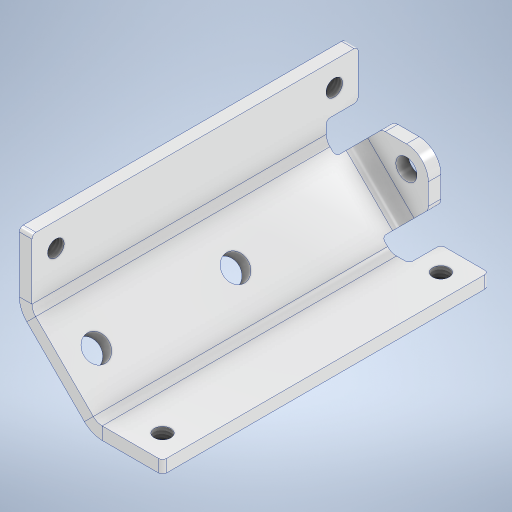
# Autodesk Inventor part: Exterior Frame Gantry Brace
Saved by Autodesk Inventor 2024 (Build 280153000, 153)
## iProperties
Created: 2024-12-02
Part Number: Exterior Frame Gantry Brace
Material: Aluminum 6061
Document SubType Name: Sheet Metal
Designer: Ishaan
Density: 2.7 g/cm^3
Sheet Metal Rule: SendCutSend_1-8_Alu
Appearance: Aluminum - Flat
Author: Ishaan
Autodesk Inventor part; units mm, degrees
ref_plane "YZ Plane" through (0, 0, 0) normal (1, 0, 0) x (0, 1, 0)
ref_plane "XZ Plane" through (0, 0, 0) normal (0, 1, 0) x (-1, 0, 0)
ref_plane "XY Plane" through (0, 0, 0) normal (0, 0, 1) x (1, 0, 0)
sketch "Sketch1" plane through (0, 0, 0) normal (0, 0, 1) x (1, 0, 0)
  line L0 (0, -21.2132) -> (-21.2132, 0) construction
  line L1 (-21.2132, 0) -> (0, 21.2132) construction
  line L2 (0, 21.2132) -> (21.2132, 0) construction
  line L3 (21.2132, 0) -> (0, -21.2132) construction
  line L4 (0, -21.2132) -> (0, 21.2132) construction
  line L5 (-21.2132, 0) -> (21.2132, 0) construction
  line L6 (42.4264, -1.5) -> (0, -1.5) construction
  line L7 (0, -1.5) -> (0, 1.5) construction
  line L8 (0, 1.5) -> (42.4264, 1.5) construction
  line L9 (42.4264, 1.5) -> (42.4264, -1.5) construction
  line L10 (42.4264, -1.5) -> (0, 1.5) construction
  line L11 (0, -1.5) -> (42.4264, 1.5) construction
  line L12 (-1.5, 42.4264) -> (1.5, 42.4264) construction
  line L13 (1.5, 42.4264) -> (1.5, 0) construction
  line L14 (1.5, 0) -> (-1.5, 0) construction
  line L15 (-1.5, 0) -> (-1.5, 42.4264) construction
  line L16 (-1.5, 42.4264) -> (1.5, 0) construction
  line L17 (1.5, 42.4264) -> (-1.5, 0) construction
  line L18 (31.5, 1.5) -> (31.5, -7.4041) construction
  line L19 (1.5, 31.5) -> (-12.6446, 31.5) construction
  line L20 (24, 1.5) -> (24, -1.5) construction
  line L21 (37.5, 1.5) -> (19.7132, 1.5)
  line L22 (19.7132, 1.5) -> (1.5, 19.7132)
  line L23 (1.5, 19.7132) -> (1.5, 37.5)
  point P0 (0, 0)
  point P1 (0, 0)
  point P2 (0, 0)
  point P3 (0, 0)
  dimension "d0" = 30
  dimension "d1" = 3
  dimension "d2" = 3
  dimension "d4" = 31.5
  dimension "d5" = 31.5
  dimension "d6" = 24
  dimension "d7" = 7.5
  dimension "d18" = 6
  dimension "d19" = 6
  measures "d0" distance of L0.end L1.end
  measures "d1" distance of L6.end L7.end
  measures "d2" distance of L13.end L14.end
  measures "d4" distance from line of L18 point (0, 0)
  measures "d5" distance from line of point (0, 0) L19
  measures "d6" distance from line of point (0, 0) L20
  measures "d7" distance between parallel lines of L20 L18
  measures "d18" distance from line of L23.end L19
  measures "d19" distance from line of L21.start L18
contour flange "Contour Flange1" sketch "Sketch1" thickness 3.175 bend radius 3.175 width 82 along (0, 0, 1) mid plane no both sides no wall seen from (28.6066, 1.5, 0) lies toward (0, 1, 0) curves L21 L22 L23
bend "Bend2"
corner "Corner1"
sketch "Sketch4" plane through (37.5, 4.675, 82) normal (0, 1, 0) x (1, 0, 0)
  line L0 (-6, 76) -> (-6, 6) construction
  line L1 (-15.1565, 0) -> (-15.1565, 82) projected
  line L2 (0, 0) -> (-15.1565, 0) projected
  line L3 (0, 82) -> (0, 0) projected
  line L4 (0, 82) -> (-15.1565, 82) projected
  circle A0 centre (-6, 6) radius 6
  line L5 (0, 0) -> (-15.1565, 0) projected
  line L6 (0, 82) -> (0, 0) projected
  circle A1 centre (-6, 76) radius 6
  line L7 (0, 82) -> (-15.1565, 82) projected
  point P0 (-37.5, 82)
  point P1 (-6, 82)
  point P2 (-6, 82)
  point P3 (-6, 82)
  point P4 (-6, 82)
  point P5 (0, 76)
  point P6 (0, 6)
  point P7 (-6, 0)
  dimension "d76" = 70
  constraints: 5 tangent, 2 centre point, 2 coincident, 2 end point, 1 point on line, 1 vertical
  measures "d76" distance of L0.start L0.end
hole "Hole1" at (31.5, 4.675, 76) at (31.5, 4.675, 6) direction (0, -1, 0) diameter 4.134 end through all thread size "M5x0.8" class "6H" standard "ANSI Metric M Profile"
sketch "Sketch5" plane through (4.675, 37.5, 82) normal (1, 0, 0) x (0, 0, -1)
  line L0 (6, -6) -> (76, -6) construction
  line L1 (0, -15.1565) -> (82, -15.1565) projected
  line L2 (82, -15.1565) -> (82, 0) projected
  line L3 (82, 0) -> (0, 0) projected
  line L4 (0, -15.1565) -> (0, 0) projected
  circle A0 centre (6, -6) radius 6
  line L5 (82, 0) -> (0, 0) projected
  line L6 (0, -15.1565) -> (0, 0) projected
  circle A1 centre (76, -6) radius 6
  line L7 (82, -15.1565) -> (82, 0) projected
  point P0 (82, -37.5)
  point P1 (82, -6)
  point P2 (82, -6)
  point P3 (82, -6)
  point P4 (76, 0)
  point P5 (82, -6)
  point P6 (0, -6)
  point P7 (6, 0)
  constraints: 4 tangent, 2 centre point, 2 coincident, 2 end point, 1 horizontal, 1 point on line
hole "Hole2" at (4.675, 31.5, 6) at (4.675, 31.5, 76) direction (-1, 0, 0) diameter 4.134 end through all thread size "M5x0.8" class "6H" standard "ANSI Metric M Profile"
sketch "Sketch6" plane through (4.675, 22.3435, 0) normal (0, 0, -1) x (-1, 0, 0)
  line L0 (-32.825, -17.6685) -> (-17.6685, -17.6685) projected
  line L1 (-15.4234, -16.7385) -> (-13.1783, -18.9836) projected
  arc A0 (-17.6685, -17.6685) -> (-15.4234, -16.7385) centre (-17.6685, -14.4935) ccw projected
  line L2 (-17.6685, -17.6685) -> (-17.6685, -20.8435) construction
  arc A1 (-17.6685, -20.8435) -> (-13.1783, -18.9836) centre (-17.6685, -14.4935) ccw projected
  line L3 (-0.9299, -2.2451) -> (1.3151, -4.4901) projected
  line L4 (-15.4234, -16.7385) -> (-0.9299, -2.2451) projected
  line L5 (-15.4234, -16.7385) -> (-13.1783, -18.9836) projected
  line L6 (-13.1783, -18.9836) -> (1.3151, -4.4901) projected
  line L7 (0, 0) -> (3.175, 0) projected
  arc A2 (-0.9299, -2.2451) -> (0, 0) centre (-3.175, 0) ccw projected
  line L8 (-0.9299, -2.2451) -> (1.3151, -4.4901) projected
  arc A3 (1.3151, -4.4901) -> (3.175, 0) centre (-3.175, 0) ccw projected
  line L9 (0, 0) -> (0, 15.1565) projected
  line L10 (0, 0) -> (3.175, 0) projected
  line L11 (3.175, 0) -> (3.175, 15.1565) projected
  line L12 (-32.825, -20.8435) -> (-17.6685, -20.8435) projected
  line L13 (-17.6685, -17.6685) -> (-17.6685, -20.8435) projected
  line L14 (-32.825, -17.6685) -> (-17.6685, -17.6685) projected
  line L15 (-20.825, -17.6685) -> (-20.825, -20.8435)
  line L16 (-14.0092, -15.3243) -> (-11.7641, -17.5694)
  line L17 (-2.3441, -3.6593) -> (-0.0991, -5.9043)
  line L18 (0, 3.1565) -> (3.175, 3.1565)
  line L19 (-15.4234, -16.7385) -> (-13.1783, -18.9836) projected
  line L20 (-32.825, -17.6685) -> (-32.825, -20.8435) projected
  line L21 (0, 15.1565) -> (3.175, 15.1565) projected
  line L22 (-26.825, -20.8435) -> (-26.825, -29.7476) construction
  line L23 (3.175, 9.1565) -> (17.3196, 9.1565) construction
  point P0 (4.675, -22.3435)
  point P1 (-17.6685, -17.6685)
  point P2 (-17.6685, -20.8435)
  dimension "d49" = 2
  dimension "d50" = 2
  dimension "d55" = 6
  dimension "d56" = 6
  constraints: 8 end point, 8 point on line, 4 perpendicular, 1 parallel
  measures "d49" distance between parallel lines of L3 L17
  measures "d50" distance between parallel lines of L16 L1
  measures "d55" distance between parallel lines of L23 L18
  measures "d56" distance between parallel lines of L22 L15
extrude "Extrusion3" cut sketch "Sketch6" against normal blind 8 contours L0 L13 L12 L15 | A0 L1 A1 L13 | L4 L16 L6 L1 | L4 L3 L6 L17 | A2 L7 A3 L3 | L9 L18 L11 L7
fillet "Fillet1" radius 1 10 edges at (5.8966, 17.5616, 8) (17.5616, 5.8966, 8) (25.5, 3.0875, 8) (3.0875, 25.5, 8) (3.0875, 25.5, 0) (25.5, 3.0875, 0) (37.5, 3.0875, 82) (37.5, 3.0875, 0) (3.0875, 37.5, 0) (3.0875, 37.5, 82)
sketch "Sketch9" plane through (18.6842, 7.0191, 0) normal (0, 0, -1) x (-0.7071068, -0.7071068, 0)
  point P0 (18.175, 8.2484)
sketch "Sketch10" plane through (5.6049, 20.0984, 8) normal (0.7071068, 0.7071068, 0) x (-0.7071068, 0.7071068, 0)
  line L0 (-18.4968, -8) -> (-2, -8)
  line L1 (-18.4968, -8) -> (-2, -8)
  line L2 (-2, -8) -> (-2, -9)
  line L3 (-2, -9) -> (-18.4968, -9)
  line L4 (-18.4968, -9) -> (-18.4968, -8)
  point P0 (-10.2484, -8)
  dimension "d77" = 1
  measures "d77" distance of L0.end L2.end
sheet face with bend "Face3" sketch "Sketch10" thickness 3.175 toward (-0.7071068, -0.7071068, 0) bend radius 3.175
bend "Bend4"
sketch "Sketch7" plane through (4.7741, 16.4391, 2.175) normal (0, 0, -1) x (-1, 0, 0)
  line L0 (-11.665, -11.665) -> (0, 0)
  line L1 (0, 0) -> (-12.4981, 12.4981)
  line L2 (-12.4981, 12.4981) -> (-24.1631, 0.8331)
  line L3 (-24.1631, 0.8331) -> (-11.665, -11.665)
  constraints: 6 end point, 1 perpendicular, 2 other
edge flange "Flange1" height 14.5 angle 90 thickness 3.175 bend radius 3.175 thickness toward (0, 0, -1) relief tear relief width 3.175 relief depth 1.5875 edges at (12.8517, 12.8517, -1) wall of the first edge with corners at (16.4391, 4.7741, 2.175) (4.7741, 16.4391, 2.175) (17.2722, 28.9372, 2.175) (28.9372, 17.2722, 2.175)
bend "Bend3"
corner "Corner2"
sketch "Sketch8" plane through (5.6049, 20.0984, 8) normal (0.7071068, 0.7071068, 0) x (-0.7071068, 0.7071068, 0)
  line L0 (-10.2484, 66) -> (-10.2484, 31) construction
  line L1 (-20.4968, 74) -> (0, 74) projected
  point P0 (-10.2484, -8)
  point P1 (-10.2484, 74)
  dimension "d67" = 35
  dimension "d68" = 8
  constraints: 2 coincident, 2 end point, 1 midpoint, 1 point on line, 1 vertical
  measures "d67" distance of L0.start L0.end
  measures "d68" distance from line of L1 L0.start
hole "Hole3" at (12.8517, 12.8517, 74) at (12.8517, 12.8517, 39) direction (-0.7071068, -0.7071068, 0) diameter 6.3 end through all
sketch "Sketch11" plane through (28.9372, 17.2722, 2.175) normal (0, 0, 1) x (0.7071068, 0.7071068, 0)
  line L0 (-11.325, 16.4968) -> (-11.325, 0) projected
  line L1 (-11.325, 0) -> (0, 0) projected
  line L2 (0, 0) -> (0, 16.4968) projected
  line L3 (-11.325, 16.4968) -> (0, 16.4968) projected
  circle A0 centre (-5.8049, 8.2484) radius 5.5
  line L4 (0, 0) -> (0, 16.4968) projected
  line L5 (-1.9159, 4.3593) -> (-6.2752, 0)
  line L6 (-1.9159, 12.1375) -> (-6.2752, 16.4968)
  line L7 (-15.8151, -6.4901) -> (-5.8049, -16.5003) projected
  point P0 (-32.675, 8.2484)
  point P1 (0, 8.2484)
  point P2 (0, 6.1839)
  dimension "d83" = 11
  dimension "d94" = 17.5
  constraints: 4 end point, 2 point on circle, 2 point on line, 2 tangent, 1 centre point, 1 horizontal alignment, 1 midpoint, 1 perpendicular, 1 vertical alignment
  measures "d83" diameter of A0
  measures "d94" distance from line of L7 A0.centre
extrude "Extrusion4" cut sketch "Sketch11" against normal through all contours L3 L2 L1 L5 A0 L6
fillet "Fillet2" radius 2 2 edges at (12.835, 24.5, 0.5875) (24.5, 12.835, 0.5875)
hole "Hole4" at (19, 19, 2.175) direction (0, 0, -1) diameter 5.3 end through all
equation "\"d4\" = d5"
equation "\"d19\" = d18"
equation "\"d35\" = Thickness"
equation "\"d49\" = d48"
equation "\"d50\" = d49"
equation "\"d55\" = d18"
equation "\"d56\" = d19"
equation "\"d10\" = Thickness"
equation "\"d20\" = BendReliefWidth"
equation "\"d21\" = BendReliefDepth"
equation "\"d22\" = MinimumRemnant"
equation "\"d23\" = TransitionRadius"
equation "\"d25\" = BendRadius"
equation "\"d27\" = CornerReliefSize"
equation "\"d28\" = GapSize"
equation "\"d29\" = JacobiRadiusSize"
equation "\"d57\" = BendReliefWidth"
equation "\"d58\" = BendReliefDepth"
equation "\"d59\" = MinimumRemnant"
equation "\"d60\" = TransitionRadius"
equation "\"d63\" = BendRadius"
equation "\"d64\" = CornerReliefSize"
equation "\"d65\" = GapSize"
equation "\"d66\" = JacobiRadiusSize"
equation "\"d78\" = BendRadius"
equation "\"d79\" = BendReliefWidth"
equation "\"d81\" = MinimumRemnant"
equation "\"d80\" = BendReliefDepth"
equation "\"d82\" = TransitionRadius"
equation "\"BendReliefWidth\" = Thickness"
equation "\"BendReliefDepth\" = 0.5 * Thickness"
equation "\"CornerReliefSize\" = 4 * Thickness"
equation "\"MinimumRemnant\" = 2 * Thickness"
equation "\"TransitionRadius\" = BendRadius"
equation "\"JacobiRadiusSize\" = BendRadius"
equation "\"GapSize\" = Thickness"
equation "\"Thickness\" = 3.175"
equation "\"d48\" = 2"
equation "\"BendRadius\" = 3.175"
body "Solid1"
